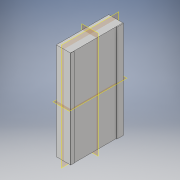
# Autodesk Inventor part: TAZ 6 Convex Model
Saved by Autodesk Inventor 2019 (Build 230136000, 136)
## iProperties
Created: 2021-02-10
Part Number: TAZ 6 Convex Model
Material: Generic
Document SubType Name: Modeling
Designer: Eric
Density: 1 g/cm^3
Appearance: Default
Author: Eric
Autodesk Inventor part; units mm, degrees
ref_plane "YZ Plane" through (0, 0, 0) normal (1, 0, 0) x (0, 1, 0)
ref_plane "XZ Plane" through (0, 0, 0) normal (0, 1, 0) x (-1, 0, 0)
ref_plane "XY Plane" through (0, 0, 0) normal (0, 0, 1) x (1, 0, 0)
sketch "Sketch7" plane through (0, 0, 0) normal (0, 1, 0) x (-1, 0, 0)
  line L0 (0, 0) -> (96.005, 0)
  line L1 (96.005, 0) -> (96.005, 353.434)
  line L2 (96.005, 353.434) -> (0, 353.434)
  line L3 (0, 353.434) -> (0, 0)
  dimension "d17" = 353.434
  dimension "d18" = 96.005
  constraints: 8 end point, 2 horizontal, 2 vertical
  measures "d17" distance of L2.end L0.start
  measures "d18" distance of L1.end L2.end
extrude "Extrusion5" add sketch "Sketch7" along normal blind 655
sketch "Sketch8" plane through (0, 0, 353.434) normal (1, 0, 0) x (0, 0, -1)
  line L0 (0, 0) -> (353.434, 0) projected
  line L1 (353.434, 0) -> (353.434, 655) projected
  line L2 (0, 655) -> (353.434, 655) projected
  line L3 (0, 0) -> (0, 655) projected
  line L4 (353.434, 655) -> (308, 655)
  line L5 (308, 655) -> (308, 0)
  line L6 (308, 0) -> (353.434, 0)
  line L7 (22, 0) -> (0, 0)
  line L8 (0, 0) -> (0, 655)
  line L9 (0, 655) -> (22, 655)
  line L10 (22, 655) -> (22, 0)
  dimension "d21" = 45.434
  dimension "d22" = 22
  constraints: 14 end point, 4 collinear, 2 parallel, 1 point on line
  measures "d21" distance of L1.end L4.end
  measures "d22" distance of L8.end L9.end
ref_plane "Work Plane16" through (2.425, 613, 26.434) normal (1, 0, 0) x (0, 1, 0)
extrude "Extrusion6" add sketch "Sketch8" along normal up to surface (2.425 mm away) separate body contours L5 L2 L1 L0
extrude "Extrusion7" add sketch "Sketch8" along normal blind 3 from surface at 2.425 contours L5 L2 L1 L0 bodies 2
ref_plane "Work Plane17" through (1.5, 633, 331.434) normal (1, 0, 0) x (0, 1, 0)
extrude "Extrusion8" add sketch "Sketch8" along normal up to surface (1.5 mm away) separate body contours L3 L2 L10 L0
ref_plane "Work Plane18" through (-45.29, 0, 45.434) normal (1, 0, 0) x (0, 0, -1)
ref_plane "Work Plane19" through (-96.005, 0, 176.717) normal (0, 0, 1) x (1, 0, 0)
ref_plane "Work Plane20" through (0, 327.5, 0) normal (0, 1, 0) x (1, 0, 0)
body "Solid1"
body "Solid5"
body "Solid6"
body "Solid7"
